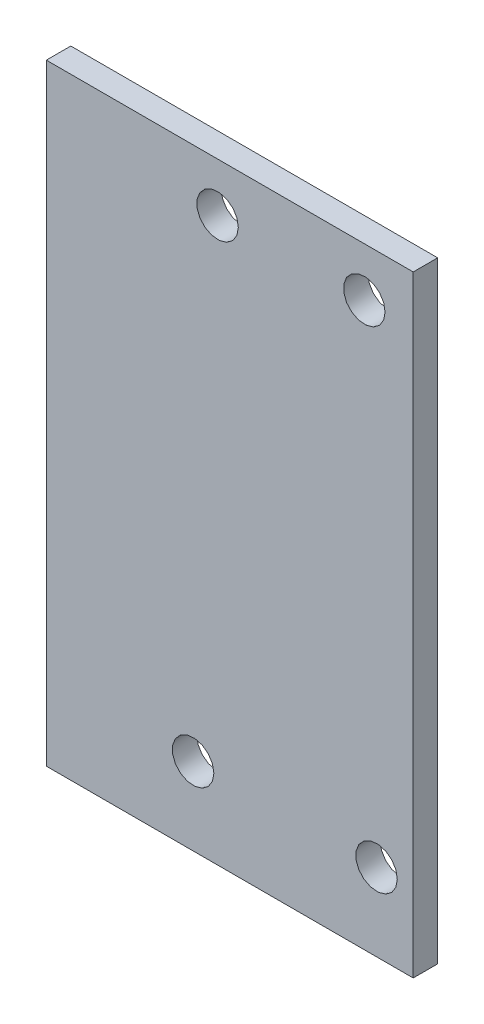
# Autodesk Inventor part: Z-head-sideplate
Saved by Autodesk Inventor 2016 (Build 200138000, 138)
## iProperties
Created: 2015-05-16
Part Number: Z-head-sideplate
Material: Aluminum 6061
Document SubType Name: Modeling
Designer: as
Mass: 7.90389 g
Surface Area: 33.3282 cm^2
Volume: 2.92737 cm^3
Density: 2.7 g/cm^3
Appearance: Aluminum - Flat
Author: as
Autodesk Inventor part; units mm, degrees
ref_plane "YZ Plane" through (0, 0, 0) normal (1, 0, 0) x (0, 1, 0)
ref_plane "XZ Plane" through (0, 0, 0) normal (0, 1, 0) x (-1, 0, 0)
ref_plane "XY Plane" through (0, 0, 0) normal (0, 0, 1) x (1, 0, 0)
sketch "Sketch1" plane through (0, 0, 0) normal (0, 0, 1) x (1, 0, 0)
  line L0 (-67.4481, -61.1843) -> (-37.4481, -61.1843)
  line L1 (-37.4481, -61.1843) -> (-37.4481, -111.1843)
  line L2 (-37.4481, -111.1843) -> (-67.4481, -111.1843)
  line L3 (-67.4481, -111.1843) -> (-67.4481, -61.1843)
  dimension "d4" = 30
  dimension "d5" = 50
  constraints: 8 end point, 2 parallel, 1 horizontal, 1 perpendicular
  measures "d4" distance of L1.end L2.end
  measures "d5" distance of L0.end L1.end
extrude "Extrusion1" add sketch "Sketch1" along normal blind 2
sketch "Sketch2" plane through (0, 0, 2) normal (0, 0, 1) x (1, 0, 0)
  point P0 (-53.4481, -65.1843)
  point P1 (-41.4481, -65.1843)
hole "Hole1" at (-53.4481, -65.1843, 2) at (-41.4481, -65.1843, 2) direction (0, 0, -1) diameter 3.4 depth 2
sketch "Sketch3" plane through (0, 0, 2) normal (0, 0, 1) x (1, 0, 0)
  point P0 (-40.4481, -104.8443)
  point P1 (-55.4481, -104.8443)
hole "Hole3" at (-40.4481, -104.8443, 2) at (-55.4481, -104.8443, 2) direction (0, 0, -1) diameter 3.4 depth 2
body "Solid1"
